Autodesk Fusion 360 part; units mm, degrees
(part 2 of 14)
  line L872 (-87.0011, -128.5875) -> (-81.5018, -138.1125)
  line L873 (-81.5018, -119.0625) -> (-87.0011, -128.5875)
  line L874 (-100.7493, -149.225) -> (-89.7507, -149.225)
  line L875 (-89.7507, -149.225) -> (-84.2515, -139.7)
  line L876 (-84.2515, -139.7) -> (-89.7507, -130.175)
  line L877 (-89.7507, -130.175) -> (-100.7493, -130.175)
  line L878 (-106.2485, -139.7) -> (-100.7493, -149.225)
  line L879 (-100.7493, -130.175) -> (-106.2485, -139.7)
  line L880 (-119.9967, -160.3375) -> (-108.9982, -160.3375)
  line L881 (-108.9982, -160.3375) -> (-103.4989, -150.8125)
  line L882 (-103.4989, -150.8125) -> (-108.9982, -141.2875)
  line L883 (-108.9982, -141.2875) -> (-119.9967, -141.2875)
  line L884 (-125.4959, -150.8125) -> (-119.9967, -160.3375)
  line L885 (-119.9967, -141.2875) -> (-125.4959, -150.8125)
  line L886 (-139.2441, -171.45) -> (-128.2456, -171.45)
  line L887 (-128.2456, -171.45) -> (-122.7463, -161.925)
  line L888 (-122.7463, -161.925) -> (-128.2456, -152.4)
  line L889 (-128.2456, -152.4) -> (-139.2441, -152.4)
  line L890 (-144.7434, -161.925) -> (-139.2441, -171.45)
  line L891 (-139.2441, -152.4) -> (-144.7434, -161.925)
  line L892 (-158.4915, -182.5625) -> (-147.493, -182.5625)
  line L893 (-147.493, -182.5625) -> (-141.9937, -173.0375)
  line L894 (-141.9937, -173.0375) -> (-147.493, -163.5125)
  line L895 (-147.493, -163.5125) -> (-158.4915, -163.5125)
  line L896 (-163.9908, -173.0375) -> (-158.4915, -182.5625)
  line L897 (-158.4915, -163.5125) -> (-163.9908, -173.0375)
  line L898 (-177.7389, -193.675) -> (-166.7404, -193.675)
  line L899 (-166.7404, -193.675) -> (-161.2411, -184.15)
  line L900 (-161.2411, -184.15) -> (-166.7404, -174.625)
  line L901 (-166.7404, -174.625) -> (-177.7389, -174.625)
  line L902 (-183.2382, -184.15) -> (-177.7389, -193.675)
  line L903 (-177.7389, -174.625) -> (-183.2382, -184.15)
  line L904 (-196.9863, -204.7875) -> (-185.9878, -204.7875)
  line L905 (-185.9878, -204.7875) -> (-180.4886, -195.2625)
  line L906 (-180.4886, -195.2625) -> (-185.9878, -185.7375)
  line L907 (-185.9878, -185.7375) -> (-196.9863, -185.7375)
  line L908 (-202.4856, -195.2625) -> (-196.9863, -204.7875)
  line L909 (-196.9863, -185.7375) -> (-202.4856, -195.2625)
  line L910 (91.7249, -60.325) -> (102.7234, -60.325)
  line L911 (102.7234, -60.325) -> (108.2227, -50.8)
  line L912 (108.2227, -50.8) -> (102.7234, -41.275)
  line L913 (102.7234, -41.275) -> (91.7249, -41.275)
  line L914 (86.2256, -50.8) -> (91.7249, -60.325)
  line L915 (91.7249, -41.275) -> (86.2256, -50.8)
  line L916 (72.4775, -71.4375) -> (83.476, -71.4375)
  line L917 (83.476, -71.4375) -> (88.9753, -61.9125)
  line L918 (88.9753, -61.9125) -> (83.476, -52.3875)
  line L919 (83.476, -52.3875) -> (72.4775, -52.3875)
  line L920 (66.9782, -61.9125) -> (72.4775, -71.4375)
  line L921 (72.4775, -52.3875) -> (66.9782, -61.9125)
  line L922 (53.2301, -82.55) -> (64.2286, -82.55)
  line L923 (64.2286, -82.55) -> (69.7278, -73.025)
  line L924 (69.7278, -73.025) -> (64.2286, -63.5)
  line L925 (64.2286, -63.5) -> (53.2301, -63.5)
  line L926 (47.7308, -73.025) -> (53.2301, -82.55)
  line L927 (53.2301, -63.5) -> (47.7308, -73.025)
  line L928 (33.9826, -93.6625) -> (44.9812, -93.6625)
  line L929 (44.9812, -93.6625) -> (50.4804, -84.1375)
  line L930 (50.4804, -84.1375) -> (44.9812, -74.6125)
  line L931 (44.9812, -74.6125) -> (33.9826, -74.6125)
  line L932 (28.4834, -84.1375) -> (33.9826, -93.6625)
  line L933 (33.9826, -74.6125) -> (28.4834, -84.1375)
  line L934 (14.7352, -104.775) -> (25.7337, -104.775)
  line L935 (25.7337, -104.775) -> (31.233, -95.25)
  line L936 (31.233, -95.25) -> (25.7337, -85.725)
  line L937 (25.7337, -85.725) -> (14.7352, -85.725)
  line L938 (9.236, -95.25) -> (14.7352, -104.775)
  line L939 (14.7352, -85.725) -> (9.236, -95.25)
  line L940 (-4.5122, -115.8875) -> (6.4863, -115.8875)
  line L941 (6.4863, -115.8875) -> (11.9856, -106.3625)
  line L942 (11.9856, -106.3625) -> (6.4863, -96.8375)
  line L943 (6.4863, -96.8375) -> (-4.5122, -96.8375)
  line L944 (-10.0114, -106.3625) -> (-4.5122, -115.8875)
  line L945 (-4.5122, -96.8375) -> (-10.0114, -106.3625)
  line L946 (-23.7596, -127) -> (-12.7611, -127)
  line L947 (-12.7611, -127) -> (-7.2618, -117.475)
  line L948 (-7.2618, -117.475) -> (-12.7611, -107.95)
  line L949 (-12.7611, -107.95) -> (-23.7596, -107.95)
  line L950 (-29.2589, -117.475) -> (-23.7596, -127)
  line L951 (-23.7596, -107.95) -> (-29.2589, -117.475)
  line L952 (-43.007, -138.1125) -> (-32.0085, -138.1125)
  line L953 (-32.0085, -138.1125) -> (-26.5092, -128.5875)
  line L954 (-26.5092, -128.5875) -> (-32.0085, -119.0625)
  line L955 (-32.0085, -119.0625) -> (-43.007, -119.0625)
  line L956 (-48.5063, -128.5875) -> (-43.007, -138.1125)
  line L957 (-43.007, -119.0625) -> (-48.5063, -128.5875)
  line L958 (-62.2544, -149.225) -> (-51.2559, -149.225)
  line L959 (-51.2559, -149.225) -> (-45.7566, -139.7)
  line L960 (-45.7566, -139.7) -> (-51.2559, -130.175)
  line L961 (-51.2559, -130.175) -> (-62.2544, -130.175)
  line L962 (-67.7537, -139.7) -> (-62.2544, -149.225)
  line L963 (-62.2544, -130.175) -> (-67.7537, -139.7)
  line L964 (-81.5018, -160.3375) -> (-70.5033, -160.3375)
  line L965 (-70.5033, -160.3375) -> (-65.0041, -150.8125)
  line L966 (-65.0041, -150.8125) -> (-70.5033, -141.2875)
  line L967 (-70.5033, -141.2875) -> (-81.5018, -141.2875)
  line L968 (-87.0011, -150.8125) -> (-81.5018, -160.3375)
  line L969 (-81.5018, -141.2875) -> (-87.0011, -150.8125)
  line L970 (-100.7493, -171.45) -> (-89.7507, -171.45)
  line L971 (-89.7507, -171.45) -> (-84.2515, -161.925)
  line L972 (-84.2515, -161.925) -> (-89.7507, -152.4)
  line L973 (-89.7507, -152.4) -> (-100.7493, -152.4)
  line L974 (-106.2485, -161.925) -> (-100.7493, -171.45)
  line L975 (-100.7493, -152.4) -> (-106.2485, -161.925)
  line L976 (-119.9967, -182.5625) -> (-108.9982, -182.5625)
  line L977 (-108.9982, -182.5625) -> (-103.4989, -173.0375)
  line L978 (-103.4989, -173.0375) -> (-108.9982, -163.5125)
  line L979 (-108.9982, -163.5125) -> (-119.9967, -163.5125)
  line L980 (-125.4959, -173.0375) -> (-119.9967, -182.5625)
  line L981 (-119.9967, -163.5125) -> (-125.4959, -173.0375)
  line L982 (-139.2441, -193.675) -> (-128.2456, -193.675)
  line L983 (-128.2456, -193.675) -> (-122.7463, -184.15)
  line L984 (-122.7463, -184.15) -> (-128.2456, -174.625)
  line L985 (-128.2456, -174.625) -> (-139.2441, -174.625)
  line L986 (-144.7434, -184.15) -> (-139.2441, -193.675)
  line L987 (-139.2441, -174.625) -> (-144.7434, -184.15)
  line L988 (-158.4915, -204.7875) -> (-147.493, -204.7875)
  line L989 (-147.493, -204.7875) -> (-141.9937, -195.2625)
  line L990 (-141.9937, -195.2625) -> (-147.493, -185.7375)
  line L991 (-147.493, -185.7375) -> (-158.4915, -185.7375)
  line L992 (-163.9908, -195.2625) -> (-158.4915, -204.7875)
  line L993 (-158.4915, -185.7375) -> (-163.9908, -195.2625)
  line L994 (-177.7389, -215.9) -> (-166.7404, -215.9)
  line L995 (-166.7404, -215.9) -> (-161.2411, -206.375)
  line L996 (-161.2411, -206.375) -> (-166.7404, -196.85)
  line L997 (-166.7404, -196.85) -> (-177.7389, -196.85)
  line L998 (-183.2382, -206.375) -> (-177.7389, -215.9)
  line L999 (-177.7389, -196.85) -> (-183.2382, -206.375)
  line L1000 (110.9723, -71.4375) -> (121.9708, -71.4375)
  line L1001 (121.9708, -71.4375) -> (127.4701, -61.9125)
  line L1002 (127.4701, -61.9125) -> (121.9708, -52.3875)
  line L1003 (121.9708, -52.3875) -> (110.9723, -52.3875)
  line L1004 (105.473, -61.9125) -> (110.9723, -71.4375)
  line L1005 (110.9723, -52.3875) -> (105.473, -61.9125)
  line L1006 (91.7249, -82.55) -> (102.7234, -82.55)
  line L1007 (102.7234, -82.55) -> (108.2227, -73.025)
  line L1008 (108.2227, -73.025) -> (102.7234, -63.5)
  line L1009 (102.7234, -63.5) -> (91.7249, -63.5)
  line L1010 (86.2256, -73.025) -> (91.7249, -82.55)
  line L1011 (91.7249, -63.5) -> (86.2256, -73.025)
  line L1012 (72.4775, -93.6625) -> (83.476, -93.6625)
  line L1013 (83.476, -93.6625) -> (88.9753, -84.1375)
  line L1014 (88.9753, -84.1375) -> (83.476, -74.6125)
  line L1015 (83.476, -74.6125) -> (72.4775, -74.6125)
  line L1016 (66.9782, -84.1375) -> (72.4775, -93.6625)
  line L1017 (72.4775, -74.6125) -> (66.9782, -84.1375)
  line L1018 (53.2301, -104.775) -> (64.2286, -104.775)
  line L1019 (64.2286, -104.775) -> (69.7278, -95.25)
  line L1020 (69.7278, -95.25) -> (64.2286, -85.725)
  line L1021 (64.2286, -85.725) -> (53.2301, -85.725)
  line L1022 (47.7308, -95.25) -> (53.2301, -104.775)
  line L1023 (53.2301, -85.725) -> (47.7308, -95.25)
  line L1024 (33.9826, -115.8875) -> (44.9812, -115.8875)
  line L1025 (44.9812, -115.8875) -> (50.4804, -106.3625)
  line L1026 (50.4804, -106.3625) -> (44.9812, -96.8375)
  line L1027 (44.9812, -96.8375) -> (33.9826, -96.8375)
  line L1028 (28.4834, -106.3625) -> (33.9826, -115.8875)
  line L1029 (33.9826, -96.8375) -> (28.4834, -106.3625)
  line L1030 (14.7352, -127) -> (25.7337, -127)
  line L1031 (25.7337, -127) -> (31.233, -117.475)
  line L1032 (31.233, -117.475) -> (25.7337, -107.95)
  line L1033 (25.7337, -107.95) -> (14.7352, -107.95)
  line L1034 (9.236, -117.475) -> (14.7352, -127)
  line L1035 (14.7352, -107.95) -> (9.236, -117.475)
  line L1036 (-4.5122, -138.1125) -> (6.4863, -138.1125)
  line L1037 (6.4863, -138.1125) -> (11.9856, -128.5875)
  line L1038 (11.9856, -128.5875) -> (6.4863, -119.0625)
  line L1039 (6.4863, -119.0625) -> (-4.5122, -119.0625)
  line L1040 (-10.0114, -128.5875) -> (-4.5122, -138.1125)
  line L1041 (-4.5122, -119.0625) -> (-10.0114, -128.5875)
  line L1042 (-23.7596, -149.225) -> (-12.7611, -149.225)
  line L1043 (-12.7611, -149.225) -> (-7.2618, -139.7)
  line L1044 (-7.2618, -139.7) -> (-12.7611, -130.175)
  line L1045 (-12.7611, -130.175) -> (-23.7596, -130.175)
  line L1046 (-29.2589, -139.7) -> (-23.7596, -149.225)
  line L1047 (-23.7596, -130.175) -> (-29.2589, -139.7)
  line L1048 (-43.007, -160.3375) -> (-32.0085, -160.3375)
  line L1049 (-32.0085, -160.3375) -> (-26.5092, -150.8125)
  line L1050 (-26.5092, -150.8125) -> (-32.0085, -141.2875)
  line L1051 (-32.0085, -141.2875) -> (-43.007, -141.2875)
  line L1052 (-48.5063, -150.8125) -> (-43.007, -160.3375)
  line L1053 (-43.007, -141.2875) -> (-48.5063, -150.8125)
  line L1054 (-62.2544, -171.45) -> (-51.2559, -171.45)
  line L1055 (-51.2559, -171.45) -> (-45.7566, -161.925)
  line L1056 (-45.7566, -161.925) -> (-51.2559, -152.4)
  line L1057 (-51.2559, -152.4) -> (-62.2544, -152.4)
  line L1058 (-67.7537, -161.925) -> (-62.2544, -171.45)
  line L1059 (-62.2544, -152.4) -> (-67.7537, -161.925)
  line L1060 (-81.5018, -182.5625) -> (-70.5033, -182.5625)
  line L1061 (-70.5033, -182.5625) -> (-65.0041, -173.0375)
  line L1062 (-65.0041, -173.0375) -> (-70.5033, -163.5125)
  line L1063 (-70.5033, -163.5125) -> (-81.5018, -163.5125)
  line L1064 (-87.0011, -173.0375) -> (-81.5018, -182.5625)
  line L1065 (-81.5018, -163.5125) -> (-87.0011, -173.0375)
  line L1066 (-100.7493, -193.675) -> (-89.7507, -193.675)
  line L1067 (-89.7507, -193.675) -> (-84.2515, -184.15)
  line L1068 (-84.2515, -184.15) -> (-89.7507, -174.625)
  line L1069 (-89.7507, -174.625) -> (-100.7493, -174.625)
  line L1070 (-106.2485, -184.15) -> (-100.7493, -193.675)
  line L1071 (-100.7493, -174.625) -> (-106.2485, -184.15)
  line L1072 (-119.9967, -204.7875) -> (-108.9982, -204.7875)
  line L1073 (-108.9982, -204.7875) -> (-103.4989, -195.2625)
  line L1074 (-103.4989, -195.2625) -> (-108.9982, -185.7375)
  line L1075 (-108.9982, -185.7375) -> (-119.9967, -185.7375)
  line L1076 (-125.4959, -195.2625) -> (-119.9967, -204.7875)
  line L1077 (-119.9967, -185.7375) -> (-125.4959, -195.2625)
  line L1078 (-139.2441, -215.9) -> (-128.2456, -215.9)
  line L1079 (-128.2456, -215.9) -> (-122.7463, -206.375)
  line L1080 (-122.7463, -206.375) -> (-128.2456, -196.85)
  line L1081 (-128.2456, -196.85) -> (-139.2441, -196.85)
  line L1082 (-144.7434, -206.375) -> (-139.2441, -215.9)
  line L1083 (-139.2441, -196.85) -> (-144.7434, -206.375)
  line L1084 (-158.4915, -227.0125) -> (-147.493, -227.0125)
  line L1085 (-147.493, -227.0125) -> (-141.9937, -217.4875)
  line L1086 (-141.9937, -217.4875) -> (-147.493, -207.9625)
  line L1087 (-147.493, -207.9625) -> (-158.4915, -207.9625)
  line L1088 (-163.9908, -217.4875) -> (-158.4915, -227.0125)
  line L1089 (-158.4915, -207.9625) -> (-163.9908, -217.4875)
  line L1090 (130.2197, -82.55) -> (141.2182, -82.55)
  line L1091 (141.2182, -82.55) -> (146.7175, -73.025)
  line L1092 (146.7175, -73.025) -> (141.2182, -63.5)
  line L1093 (141.2182, -63.5) -> (130.2197, -63.5)
  line L1094 (124.7205, -73.025) -> (130.2197, -82.55)
  line L1095 (130.2197, -63.5) -> (124.7205, -73.025)
  line L1096 (110.9723, -93.6625) -> (121.9708, -93.6625)
  line L1097 (121.9708, -93.6625) -> (127.4701, -84.1375)
  line L1098 (127.4701, -84.1375) -> (121.9708, -74.6125)
  line L1099 (121.9708, -74.6125) -> (110.9723, -74.6125)
  line L1100 (105.473, -84.1375) -> (110.9723, -93.6625)
  line L1101 (110.9723, -74.6125) -> (105.473, -84.1375)
  line L1102 (91.7249, -104.775) -> (102.7234, -104.775)
  line L1103 (102.7234, -104.775) -> (108.2227, -95.25)
  line L1104 (108.2227, -95.25) -> (102.7234, -85.725)
  line L1105 (102.7234, -85.725) -> (91.7249, -85.725)
  line L1106 (86.2256, -95.25) -> (91.7249, -104.775)
  line L1107 (91.7249, -85.725) -> (86.2256, -95.25)
  line L1108 (72.4775, -115.8875) -> (83.476, -115.8875)
  line L1109 (83.476, -115.8875) -> (88.9753, -106.3625)
  line L1110 (88.9753, -106.3625) -> (83.476, -96.8375)
  line L1111 (83.476, -96.8375) -> (72.4775, -96.8375)
  line L1112 (66.9782, -106.3625) -> (72.4775, -115.8875)
  line L1113 (72.4775, -96.8375) -> (66.9782, -106.3625)
  line L1114 (53.2301, -127) -> (64.2286, -127)
  line L1115 (64.2286, -127) -> (69.7278, -117.475)
  line L1116 (69.7278, -117.475) -> (64.2286, -107.95)
  line L1117 (64.2286, -107.95) -> (53.2301, -107.95)
  line L1118 (47.7308, -117.475) -> (53.2301, -127)
  line L1119 (53.2301, -107.95) -> (47.7308, -117.475)
  line L1120 (33.9826, -138.1125) -> (44.9812, -138.1125)
  line L1121 (44.9812, -138.1125) -> (50.4804, -128.5875)
  line L1122 (50.4804, -128.5875) -> (44.9812, -119.0625)
  line L1123 (44.9812, -119.0625) -> (33.9826, -119.0625)
  line L1124 (28.4834, -128.5875) -> (33.9826, -138.1125)
  line L1125 (33.9826, -119.0625) -> (28.4834, -128.5875)
  line L1126 (14.7352, -149.225) -> (25.7337, -149.225)
  line L1127 (25.7337, -149.225) -> (31.233, -139.7)
  line L1128 (31.233, -139.7) -> (25.7337, -130.175)
  line L1129 (25.7337, -130.175) -> (14.7352, -130.175)
  line L1130 (9.236, -139.7) -> (14.7352, -149.225)
  line L1131 (14.7352, -130.175) -> (9.236, -139.7)
  line L1132 (-4.5122, -160.3375) -> (6.4863, -160.3375)
  line L1133 (6.4863, -160.3375) -> (11.9856, -150.8125)
  line L1134 (11.9856, -150.8125) -> (6.4863, -141.2875)
  line L1135 (6.4863, -141.2875) -> (-4.5122, -141.2875)
  line L1136 (-10.0114, -150.8125) -> (-4.5122, -160.3375)
  line L1137 (-4.5122, -141.2875) -> (-10.0114, -150.8125)
  line L1138 (-23.7596, -171.45) -> (-12.7611, -171.45)
  line L1139 (-12.7611, -171.45) -> (-7.2618, -161.925)
  line L1140 (-7.2618, -161.925) -> (-12.7611, -152.4)
  line L1141 (-12.7611, -152.4) -> (-23.7596, -152.4)
  line L1142 (-29.2589, -161.925) -> (-23.7596, -171.45)
  line L1143 (-23.7596, -152.4) -> (-29.2589, -161.925)
  line L1144 (-43.007, -182.5625) -> (-32.0085, -182.5625)
  line L1145 (-32.0085, -182.5625) -> (-26.5092, -173.0375)
  line L1146 (-26.5092, -173.0375) -> (-32.0085, -163.5125)
  line L1147 (-32.0085, -163.5125) -> (-43.007, -163.5125)
  line L1148 (-48.5063, -173.0375) -> (-43.007, -182.5625)
  line L1149 (-43.007, -163.5125) -> (-48.5063, -173.0375)
  line L1150 (-62.2544, -193.675) -> (-51.2559, -193.675)
  line L1151 (-51.2559, -193.675) -> (-45.7566, -184.15)
  line L1152 (-45.7566, -184.15) -> (-51.2559, -174.625)
  line L1153 (-51.2559, -174.625) -> (-62.2544, -174.625)
  line L1154 (-67.7537, -184.15) -> (-62.2544, -193.675)
  line L1155 (-62.2544, -174.625) -> (-67.7537, -184.15)
  line L1156 (-81.5018, -204.7875) -> (-70.5033, -204.7875)
  line L1157 (-70.5033, -204.7875) -> (-65.0041, -195.2625)
  line L1158 (-65.0041, -195.2625) -> (-70.5033, -185.7375)
  line L1159 (-70.5033, -185.7375) -> (-81.5018, -185.7375)
  line L1160 (-87.0011, -195.2625) -> (-81.5018, -204.7875)
  line L1161 (-81.5018, -185.7375) -> (-87.0011, -195.2625)
  line L1162 (-100.7493, -215.9) -> (-89.7507, -215.9)
  line L1163 (-89.7507, -215.9) -> (-84.2515, -206.375)
  line L1164 (-84.2515, -206.375) -> (-89.7507, -196.85)
  line L1165 (-89.7507, -196.85) -> (-100.7493, -196.85)
  line L1166 (-106.2485, -206.375) -> (-100.7493, -215.9)
  line L1167 (-100.7493, -196.85) -> (-106.2485, -206.375)
  line L1168 (-119.9967, -227.0125) -> (-108.9982, -227.0125)
  line L1169 (-108.9982, -227.0125) -> (-103.4989, -217.4875)
  line L1170 (-103.4989, -217.4875) -> (-108.9982, -207.9625)
  line L1171 (-108.9982, -207.9625) -> (-119.9967, -207.9625)
  line L1172 (-125.4959, -217.4875) -> (-119.9967, -227.0125)
  line L1173 (-119.9967, -207.9625) -> (-125.4959, -217.4875)
  line L1174 (-139.2441, -238.125) -> (-128.2456, -238.125)
  line L1175 (-128.2456, -238.125) -> (-122.7463, -228.6)
  line L1176 (-122.7463, -228.6) -> (-128.2456, -219.075)
  line L1177 (-128.2456, -219.075) -> (-139.2441, -219.075)
  line L1178 (-144.7434, -228.6) -> (-139.2441, -238.125)
  line L1179 (-139.2441, -219.075) -> (-144.7434, -228.6)
  line L1180 (149.4671, -93.6625) -> (160.4657, -93.6625)
  line L1181 (160.4657, -93.6625) -> (165.9649, -84.1375)
  line L1182 (165.9649, -84.1375) -> (160.4657, -74.6125)
  line L1183 (160.4657, -74.6125) -> (149.4671, -74.6125)
  line L1184 (143.9679, -84.1375) -> (149.4671, -93.6625)
  line L1185 (149.4671, -74.6125) -> (143.9679, -84.1375)
  line L1186 (130.2197, -104.775) -> (141.2182, -104.775)
  line L1187 (141.2182, -104.775) -> (146.7175, -95.25)
  line L1188 (146.7175, -95.25) -> (141.2182, -85.725)
  line L1189 (141.2182, -85.725) -> (130.2197, -85.725)
  line L1190 (124.7205, -95.25) -> (130.2197, -104.775)
  line L1191 (130.2197, -85.725) -> (124.7205, -95.25)
  line L1192 (110.9723, -115.8875) -> (121.9708, -115.8875)
  line L1193 (121.9708, -115.8875) -> (127.4701, -106.3625)
  line L1194 (127.4701, -106.3625) -> (121.9708, -96.8375)
  line L1195 (121.9708, -96.8375) -> (110.9723, -96.8375)
  line L1196 (105.473, -106.3625) -> (110.9723, -115.8875)
  line L1197 (110.9723, -96.8375) -> (105.473, -106.3625)
  line L1198 (91.7249, -127) -> (102.7234, -127)
  line L1199 (102.7234, -127) -> (108.2227, -117.475)
  line L1200 (108.2227, -117.475) -> (102.7234, -107.95)
  line L1201 (102.7234, -107.95) -> (91.7249, -107.95)
  line L1202 (86.2256, -117.475) -> (91.7249, -127)
  line L1203 (91.7249, -107.95) -> (86.2256, -117.475)
  line L1204 (72.4775, -138.1125) -> (83.476, -138.1125)
  line L1205 (83.476, -138.1125) -> (88.9753, -128.5875)
  line L1206 (88.9753, -128.5875) -> (83.476, -119.0625)
  line L1207 (83.476, -119.0625) -> (72.4775, -119.0625)
  line L1208 (66.9782, -128.5875) -> (72.4775, -138.1125)
  line L1209 (72.4775, -119.0625) -> (66.9782, -128.5875)
  line L1210 (53.2301, -149.225) -> (64.2286, -149.225)
  line L1211 (64.2286, -149.225) -> (69.7278, -139.7)
  line L1212 (69.7278, -139.7) -> (64.2286, -130.175)
  line L1213 (64.2286, -130.175) -> (53.2301, -130.175)
  line L1214 (47.7308, -139.7) -> (53.2301, -149.225)
  line L1215 (53.2301, -130.175) -> (47.7308, -139.7)
  line L1216 (33.9826, -160.3375) -> (44.9812, -160.3375)
  line L1217 (44.9812, -160.3375) -> (50.4804, -150.8125)
  line L1218 (50.4804, -150.8125) -> (44.9812, -141.2875)
  line L1219 (44.9812, -141.2875) -> (33.9826, -141.2875)
  line L1220 (28.4834, -150.8125) -> (33.9826, -160.3375)
  line L1221 (33.9826, -141.2875) -> (28.4834, -150.8125)
  line L1222 (14.7352, -171.45) -> (25.7337, -171.45)
  line L1223 (25.7337, -171.45) -> (31.233, -161.925)
  line L1224 (31.233, -161.925) -> (25.7337, -152.4)
  line L1225 (25.7337, -152.4) -> (14.7352, -152.4)
  line L1226 (9.236, -161.925) -> (14.7352, -171.45)
  line L1227 (14.7352, -152.4) -> (9.236, -161.925)
  line L1228 (-4.5122, -182.5625) -> (6.4863, -182.5625)
  line L1229 (6.4863, -182.5625) -> (11.9856, -173.0375)
  line L1230 (11.9856, -173.0375) -> (6.4863, -163.5125)
  line L1231 (6.4863, -163.5125) -> (-4.5122, -163.5125)
  line L1232 (-10.0114, -173.0375) -> (-4.5122, -182.5625)
  line L1233 (-4.5122, -163.5125) -> (-10.0114, -173.0375)
  line L1234 (-23.7596, -193.675) -> (-12.7611, -193.675)
  line L1235 (-12.7611, -193.675) -> (-7.2618, -184.15)
  line L1236 (-7.2618, -184.15) -> (-12.7611, -174.625)
  line L1237 (-12.7611, -174.625) -> (-23.7596, -174.625)
  line L1238 (-29.2589, -184.15) -> (-23.7596, -193.675)
  line L1239 (-23.7596, -174.625) -> (-29.2589, -184.15)
  line L1240 (-43.007, -204.7875) -> (-32.0085, -204.7875)
  line L1241 (-32.0085, -204.7875) -> (-26.5092, -195.2625)
  line L1242 (-26.5092, -195.2625) -> (-32.0085, -185.7375)
  line L1243 (-32.0085, -185.7375) -> (-43.007, -185.7375)
  line L1244 (-48.5063, -195.2625) -> (-43.007, -204.7875)
  line L1245 (-43.007, -185.7375) -> (-48.5063, -195.2625)
  line L1246 (-62.2544, -215.9) -> (-51.2559, -215.9)
  line L1247 (-51.2559, -215.9) -> (-45.7566, -206.375)
  line L1248 (-45.7566, -206.375) -> (-51.2559, -196.85)
  line L1249 (-51.2559, -196.85) -> (-62.2544, -196.85)
  line L1250 (-67.7537, -206.375) -> (-62.2544, -215.9)
  line L1251 (-62.2544, -196.85) -> (-67.7537, -206.375)
  line L1252 (-81.5018, -227.0125) -> (-70.5033, -227.0125)
  line L1253 (-70.5033, -227.0125) -> (-65.0041, -217.4875)
  line L1254 (-65.0041, -217.4875) -> (-70.5033, -207.9625)
  line L1255 (-70.5033, -207.9625) -> (-81.5018, -207.9625)
  line L1256 (-87.0011, -217.4875) -> (-81.5018, -227.0125)
  line L1257 (-81.5018, -207.9625) -> (-87.0011, -217.4875)
  line L1258 (-100.7493, -238.125) -> (-89.7507, -238.125)
  line L1259 (-89.7507, -238.125) -> (-84.2515, -228.6)
  line L1260 (-84.2515, -228.6) -> (-89.7507, -219.075)
  line L1261 (-89.7507, -219.075) -> (-100.7493, -219.075)
  line L1262 (-106.2485, -228.6) -> (-100.7493, -238.125)
  line L1263 (-100.7493, -219.075) -> (-106.2485, -228.6)
  line L1264 (-119.9967, -249.2375) -> (-108.9982, -249.2375)
  line L1265 (-108.9982, -249.2375) -> (-103.4989, -239.7125)
  line L1266 (-103.4989, -239.7125) -> (-108.9982, -230.1875)
  line L1267 (-108.9982, -230.1875) -> (-119.9967, -230.1875)
  line L1268 (-125.4959, -239.7125) -> (-119.9967, -249.2375)
  line L1269 (-119.9967, -230.1875) -> (-125.4959, -239.7125)
  line L1270 (168.7145, -104.775) -> (179.7131, -104.775)
  line L1271 (179.7131, -104.775) -> (185.2123, -95.25)
  line L1272 (185.2123, -95.25) -> (179.7131, -85.725)
  line L1273 (179.7131, -85.725) -> (168.7145, -85.725)
  line L1274 (163.2153, -95.25) -> (168.7145, -104.775)
  line L1275 (168.7145, -85.725) -> (163.2153, -95.25)
  line L1276 (149.4671, -115.8875) -> (160.4657, -115.8875)
  line L1277 (160.4657, -115.8875) -> (165.9649, -106.3625)
  line L1278 (165.9649, -106.3625) -> (160.4657, -96.8375)
  line L1279 (160.4657, -96.8375) -> (149.4671, -96.8375)
  line L1280 (143.9679, -106.3625) -> (149.4671, -115.8875)
  line L1281 (149.4671, -96.8375) -> (143.9679, -106.3625)
  line L1282 (130.2197, -127) -> (141.2182, -127)
  line L1283 (141.2182, -127) -> (146.7175, -117.475)
  line L1284 (146.7175, -117.475) -> (141.2182, -107.95)
  line L1285 (141.2182, -107.95) -> (130.2197, -107.95)
  line L1286 (124.7205, -117.475) -> (130.2197, -127)
  line L1287 (130.2197, -107.95) -> (124.7205, -117.475)
  line L1288 (110.9723, -138.1125) -> (121.9708, -138.1125)
  line L1289 (121.9708, -138.1125) -> (127.4701, -128.5875)
  line L1290 (127.4701, -128.5875) -> (121.9708, -119.0625)
  line L1291 (121.9708, -119.0625) -> (110.9723, -119.0625)
  line L1292 (105.473, -128.5875) -> (110.9723, -138.1125)
  line L1293 (110.9723, -119.0625) -> (105.473, -128.5875)
  line L1294 (91.7249, -149.225) -> (102.7234, -149.225)
  line L1295 (102.7234, -149.225) -> (108.2227, -139.7)
  line L1296 (108.2227, -139.7) -> (102.7234, -130.175)
  line L1297 (102.7234, -130.175) -> (91.7249, -130.175)
  line L1298 (86.2256, -139.7) -> (91.7249, -149.225)
  line L1299 (91.7249, -130.175) -> (86.2256, -139.7)
  line L1300 (72.4775, -160.3375) -> (83.476, -160.3375)
  line L1301 (83.476, -160.3375) -> (88.9753, -150.8125)
  line L1302 (88.9753, -150.8125) -> (83.476, -141.2875)
  line L1303 (83.476, -141.2875) -> (72.4775, -141.2875)
  line L1304 (66.9782, -150.8125) -> (72.4775, -160.3375)
  line L1305 (72.4775, -141.2875) -> (66.9782, -150.8125)
  line L1306 (53.2301, -171.45) -> (64.2286, -171.45)
  line L1307 (64.2286, -171.45) -> (69.7278, -161.925)
  line L1308 (69.7278, -161.925) -> (64.2286, -152.4)
  line L1309 (64.2286, -152.4) -> (53.2301, -152.4)
  line L1310 (47.7308, -161.925) -> (53.2301, -171.45)
  line L1311 (53.2301, -152.4) -> (47.7308, -161.925)
  line L1312 (33.9826, -182.5625) -> (44.9812, -182.5625)
  line L1313 (44.9812, -182.5625) -> (50.4804, -173.0375)
  line L1314 (50.4804, -173.0375) -> (44.9812, -163.5125)
  line L1315 (44.9812, -163.5125) -> (33.9826, -163.5125)
  line L1316 (28.4834, -173.0375) -> (33.9826, -182.5625)
  line L1317 (33.9826, -163.5125) -> (28.4834, -173.0375)
  line L1318 (14.7352, -193.675) -> (25.7337, -193.675)
  line L1319 (25.7337, -193.675) -> (31.233, -184.15)
  line L1320 (31.233, -184.15) -> (25.7337, -174.625)
  line L1321 (25.7337, -174.625) -> (14.7352, -174.625)
  line L1322 (9.236, -184.15) -> (14.7352, -193.675)
  line L1323 (14.7352, -174.625) -> (9.236, -184.15)
  line L1324 (-4.5122, -204.7875) -> (6.4863, -204.7875)
  line L1325 (6.4863, -204.7875) -> (11.9856, -195.2625)
  line L1326 (11.9856, -195.2625) -> (6.4863, -185.7375)
  line L1327 (6.4863, -185.7375) -> (-4.5122, -185.7375)
  line L1328 (-10.0114, -195.2625) -> (-4.5122, -204.7875)
  line L1329 (-4.5122, -185.7375) -> (-10.0114, -195.2625)
  line L1330 (-23.7596, -215.9) -> (-12.7611, -215.9)
  line L1331 (-12.7611, -215.9) -> (-7.2618, -206.375)
  line L1332 (-7.2618, -206.375) -> (-12.7611, -196.85)
  line L1333 (-12.7611, -196.85) -> (-23.7596, -196.85)
  line L1334 (-29.2589, -206.375) -> (-23.7596, -215.9)
  line L1335 (-23.7596, -196.85) -> (-29.2589, -206.375)
  line L1336 (-43.007, -227.0125) -> (-32.0085, -227.0125)
  line L1337 (-32.0085, -227.0125) -> (-26.5092, -217.4875)
  line L1338 (-26.5092, -217.4875) -> (-32.0085, -207.9625)
  line L1339 (-32.0085, -207.9625) -> (-43.007, -207.9625)
  line L1340 (-48.5063, -217.4875) -> (-43.007, -227.0125)
  line L1341 (-43.007, -207.9625) -> (-48.5063, -217.4875)
  line L1342 (-62.2544, -238.125) -> (-51.2559, -238.125)
  line L1343 (-51.2559, -238.125) -> (-45.7566, -228.6)
  line L1344 (-45.7566, -228.6) -> (-51.2559, -219.075)
  line L1345 (-51.2559, -219.075) -> (-62.2544, -219.075)
  line L1346 (-67.7537, -228.6) -> (-62.2544, -238.125)
  line L1347 (-62.2544, -219.075) -> (-67.7537, -228.6)
  line L1348 (-81.5018, -249.2375) -> (-70.5033, -249.2375)
  line L1349 (-70.5033, -249.2375) -> (-65.0041, -239.7125)
  line L1350 (-65.0041, -239.7125) -> (-70.5033, -230.1875)
  line L1351 (-70.5033, -230.1875) -> (-81.5018, -230.1875)
  line L1352 (-87.0011, -239.7125) -> (-81.5018, -249.2375)
  line L1353 (-81.5018, -230.1875) -> (-87.0011, -239.7125)
  line L1354 (-100.7493, -260.35) -> (-89.7507, -260.35)
  line L1355 (-89.7507, -260.35) -> (-84.2515, -250.825)
  line L1356 (-84.2515, -250.825) -> (-89.7507, -241.3)
  line L1357 (-89.7507, -241.3) -> (-100.7493, -241.3)
  line L1358 (-106.2485, -250.825) -> (-100.7493, -260.35)
  line L1359 (-100.7493, -241.3) -> (-106.2485, -250.825)
  point P0 (-95.25, -95.25)
  dimension "d8" = 9.525
  dimension "d9" = 120
  dimension "d13" = 22.225
  dimension "d14" = 22.225
  constraint coincident L1.end L2.start
  constraint coincident L0.start L3.end
  constraint coincident L2.end L3.start
  constraint coincident L0.end L1.start
  constraint midpoint L4 P0
  constraint horizontal L13
  constraint coincident P0 L12.start
  constraint coincident L6.start L12
  constraint midpoint L11 L14.end
  constraint midpoint L7 L15.end
  measures "d8" distance of P0 L11
  measures "d9" angle of L12 L13
extrude "Extrude3" cut sketch "Sketch2" against normal blind 6.35 contours L0 L1 L2 L3 L46 L47 L130 L131 L134 L136 L137 L138 L140 L141 L142 L143 L144 L145 L214 L215 L218 L220 L221 L222 L224 L225 L238 L239 L240 L241 L298 L299 L302 L304 L305 L306 L308 L309 L334 L335 L336 L337 L382 L383 L386 L388 L389 L390 L392 L393 L430 L431 L432 L433 L466 L470 L472 L473 L474 L476 L477 L526 L527 L528 L529 L562 L565 L566 L567 L622 L623 L624 L625 L658 L661 L662 L663 L712 L713 L714 L715 L748 L751 L752 L753 L808 L809 L810 L811 L844 L847 L848 L849 L899 L900 L901 L902 L903 L906 L907 L940 L943 L944 L945 L983 L984 L985 L986 L987 L990 L991 L993 L1036 L1039 L1040 L1041 L1067 L1068 L1069 L1070 L1071 L1074 L1075 L1077 L1132 L1135 L1136 L1137 L1151 L1152 L1153 L1154 L1155 L1158 L1159 L1161 L1228 L1231 L1232 L1233 L1235 L1236 L1237 L1238 L1239 L1242 L1243 L1245 L1327 L1329 keep common part
extrude "Extrude4" add sketch "Sketch1" along normal blind 69.85
fillet "Fillet1" radius 12.7 4 edges at (196.85, -6.35, 34.925) (196.85, 196.85, 34.925) (-6.35, 196.85, 34.925) (-6.35, -6.35, 34.925)
fillet "Fillet2" radius 6.35 4 edges at (190.5, 190.5, 34.925) (0, 190.5, 34.925) (0, 0, 34.925) (190.5, 0, 34.925)
sketch "Sketch3" plane through (0, 196.85, 0) normal (0, 1, 0) x (-1, 0, 0)
  line L0 (-196.85, 69.85) -> (-184.15, 69.85) construction
  line L1 (-184.15, 69.85) -> (-6.35, 69.85) construction
  line L2 (-196.85, 69.85) -> (-196.85, 0) construction
  line L3 (-184.15, 0) -> (-196.85, 0) construction
  line L4 (-184.15, 0) -> (-6.35, 0) construction
  line L5 (6.35, 0) -> (-6.35, 0) construction
  line L6 (6.35, 0) -> (6.35, 69.85) construction
  line L7 (-6.35, 69.85) -> (6.35, 69.85) construction
  line L8 (6.35, 0) -> (-196.85, 69.85) construction
  line L9 (-196.85, 0) -> (6.35, 69.85) construction
  line L10 (-95.25, 34.925) -> (-75.086, 69.85) construction
  line L11 (-95.25, 34.925) -> (-135.5779, 34.925) construction
  line L12 (-89.7507, 44.45) -> (-100.7493, 44.45)
  line L13 (-100.7493, 44.45) -> (-106.2485, 34.925)
  line L14 (-106.2485, 34.925) -> (-100.7493, 25.4)
  line L15 (-100.7493, 25.4) -> (-89.7507, 25.4)
  line L16 (-89.7507, 25.4) -> (-84.2515, 34.925)
  line L17 (-84.2515, 34.925) -> (-89.7507, 44.45)
  line L18 (-95.25, 34.925) -> (-87.0011, 39.6875) construction
  line L19 (-95.25, 34.925) -> (-103.4989, 39.6875) construction
  line L20 (-378.462, -433.3875) -> (-389.4605, -433.3875)
  line L21 (-389.4605, -433.3875) -> (-394.9597, -442.9125)
  line L22 (-394.9597, -442.9125) -> (-389.4605, -452.4375)
  line L23 (-389.4605, -452.4375) -> (-378.462, -452.4375)
  line L24 (-372.9627, -442.9125) -> (-378.462, -433.3875)
  line L25 (-378.462, -452.4375) -> (-372.9627, -442.9125)
  line L26 (-359.2145, -422.275) -> (-370.2131, -422.275)
  line L27 (-370.2131, -422.275) -> (-375.7123, -431.8)
  line L28 (-375.7123, -431.8) -> (-370.2131, -441.325)
  line L29 (-370.2131, -441.325) -> (-359.2145, -441.325)
  line L30 (-353.7153, -431.8) -> (-359.2145, -422.275)
  line L31 (-359.2145, -441.325) -> (-353.7153, -431.8)
  line L32 (-339.9671, -411.1625) -> (-350.9657, -411.1625)
  line L33 (-350.9657, -411.1625) -> (-356.4649, -420.6875)
  line L34 (-356.4649, -420.6875) -> (-350.9657, -430.2125)
  line L35 (-350.9657, -430.2125) -> (-339.9671, -430.2125)
  line L36 (-334.4679, -420.6875) -> (-339.9671, -411.1625)
  line L37 (-339.9671, -430.2125) -> (-334.4679, -420.6875)
  line L38 (-320.7197, -400.05) -> (-331.7182, -400.05)
  line L39 (-331.7182, -400.05) -> (-337.2175, -409.575)
  line L40 (-337.2175, -409.575) -> (-331.7182, -419.1)
  line L41 (-331.7182, -419.1) -> (-320.7197, -419.1)
  line L42 (-315.2205, -409.575) -> (-320.7197, -400.05)
  line L43 (-320.7197, -419.1) -> (-315.2205, -409.575)
  line L44 (-301.4723, -388.9375) -> (-312.4708, -388.9375)
  line L45 (-312.4708, -388.9375) -> (-317.9701, -398.4625)
  line L46 (-317.9701, -398.4625) -> (-312.4708, -407.9875)
  line L47 (-312.4708, -407.9875) -> (-301.4723, -407.9875)
  line L48 (-295.973, -398.4625) -> (-301.4723, -388.9375)
  line L49 (-301.4723, -407.9875) -> (-295.973, -398.4625)
  line L50 (-282.2249, -377.825) -> (-293.2234, -377.825)
  line L51 (-293.2234, -377.825) -> (-298.7227, -387.35)
  line L52 (-298.7227, -387.35) -> (-293.2234, -396.875)
  line L53 (-293.2234, -396.875) -> (-282.2249, -396.875)
  line L54 (-276.7256, -387.35) -> (-282.2249, -377.825)
  line L55 (-282.2249, -396.875) -> (-276.7256, -387.35)
  line L56 (-262.9775, -366.7125) -> (-273.976, -366.7125)
  line L57 (-273.976, -366.7125) -> (-279.4753, -376.2375)
  line L58 (-279.4753, -376.2375) -> (-273.976, -385.7625)
  line L59 (-273.976, -385.7625) -> (-262.9775, -385.7625)
  line L60 (-257.4782, -376.2375) -> (-262.9775, -366.7125)
  line L61 (-262.9775, -385.7625) -> (-257.4782, -376.2375)
  line L62 (-243.7301, -355.6) -> (-254.7286, -355.6)
  line L63 (-254.7286, -355.6) -> (-260.2278, -365.125)
  line L64 (-260.2278, -365.125) -> (-254.7286, -374.65)
  line L65 (-254.7286, -374.65) -> (-243.7301, -374.65)
  line L66 (-238.2308, -365.125) -> (-243.7301, -355.6)
  line L67 (-243.7301, -374.65) -> (-238.2308, -365.125)
  line L68 (-224.4826, -344.4875) -> (-235.4812, -344.4875)
  line L69 (-235.4812, -344.4875) -> (-240.9804, -354.0125)
  line L70 (-240.9804, -354.0125) -> (-235.4812, -363.5375)
  line L71 (-235.4812, -363.5375) -> (-224.4826, -363.5375)
  line L72 (-218.9834, -354.0125) -> (-224.4826, -344.4875)
  line L73 (-224.4826, -363.5375) -> (-218.9834, -354.0125)
  line L74 (-205.2352, -333.375) -> (-216.2337, -333.375)
  line L75 (-216.2337, -333.375) -> (-221.733, -342.9)
  line L76 (-221.733, -342.9) -> (-216.2337, -352.425)
  line L77 (-216.2337, -352.425) -> (-205.2352, -352.425)
  line L78 (-199.736, -342.9) -> (-205.2352, -333.375)
  line L79 (-205.2352, -352.425) -> (-199.736, -342.9)
  line L80 (-185.9878, -322.2625) -> (-196.9863, -322.2625)
  line L81 (-196.9863, -322.2625) -> (-202.4856, -331.7875)
  line L82 (-202.4856, -331.7875) -> (-196.9863, -341.3125)
  line L83 (-196.9863, -341.3125) -> (-185.9878, -341.3125)
  line L84 (-180.4886, -331.7875) -> (-185.9878, -322.2625)
  line L85 (-185.9878, -341.3125) -> (-180.4886, -331.7875)
  line L86 (-166.7404, -311.15) -> (-177.7389, -311.15)
  line L87 (-177.7389, -311.15) -> (-183.2382, -320.675)
  line L88 (-183.2382, -320.675) -> (-177.7389, -330.2)
  line L89 (-177.7389, -330.2) -> (-166.7404, -330.2)
  line L90 (-161.2411, -320.675) -> (-166.7404, -311.15)
  line L91 (-166.7404, -330.2) -> (-161.2411, -320.675)
  line L92 (-147.493, -300.0375) -> (-158.4915, -300.0375)
  line L93 (-158.4915, -300.0375) -> (-163.9908, -309.5625)
  line L94 (-163.9908, -309.5625) -> (-158.4915, -319.0875)
  line L95 (-158.4915, -319.0875) -> (-147.493, -319.0875)
  line L96 (-141.9937, -309.5625) -> (-147.493, -300.0375)
  line L97 (-147.493, -319.0875) -> (-141.9937, -309.5625)
  line L98 (-128.2456, -288.925) -> (-139.2441, -288.925)
  line L99 (-139.2441, -288.925) -> (-144.7434, -298.45)
  line L100 (-144.7434, -298.45) -> (-139.2441, -307.975)
  line L101 (-139.2441, -307.975) -> (-128.2456, -307.975)
  line L102 (-122.7463, -298.45) -> (-128.2456, -288.925)
  line L103 (-128.2456, -307.975) -> (-122.7463, -298.45)
  line L104 (-108.9982, -277.8125) -> (-119.9967, -277.8125)
  line L105 (-119.9967, -277.8125) -> (-125.4959, -287.3375)
  line L106 (-125.4959, -287.3375) -> (-119.9967, -296.8625)
  line L107 (-119.9967, -296.8625) -> (-108.9982, -296.8625)
  line L108 (-103.4989, -287.3375) -> (-108.9982, -277.8125)
  line L109 (-108.9982, -296.8625) -> (-103.4989, -287.3375)
  line L110 (-89.7507, -266.7) -> (-100.7493, -266.7)
  line L111 (-100.7493, -266.7) -> (-106.2485, -276.225)
  line L112 (-106.2485, -276.225) -> (-100.7493, -285.75)
  line L113 (-100.7493, -285.75) -> (-89.7507, -285.75)
  line L114 (-84.2515, -276.225) -> (-89.7507, -266.7)
  line L115 (-89.7507, -285.75) -> (-84.2515, -276.225)
  line L116 (-70.5033, -255.5875) -> (-81.5018, -255.5875)
  line L117 (-81.5018, -255.5875) -> (-87.0011, -265.1125)
  line L118 (-87.0011, -265.1125) -> (-81.5018, -274.6375)
  line L119 (-81.5018, -274.6375) -> (-70.5033, -274.6375)
  line L120 (-65.0041, -265.1125) -> (-70.5033, -255.5875)
  line L121 (-70.5033, -274.6375) -> (-65.0041, -265.1125)
  line L122 (-51.2559, -244.475) -> (-62.2544, -244.475)
  line L123 (-62.2544, -244.475) -> (-67.7537, -254)
  line L124 (-67.7537, -254) -> (-62.2544, -263.525)
  line L125 (-62.2544, -263.525) -> (-51.2559, -263.525)
  line L126 (-45.7566, -254) -> (-51.2559, -244.475)
  line L127 (-51.2559, -263.525) -> (-45.7566, -254)
  line L128 (-32.0085, -233.3625) -> (-43.007, -233.3625)
  line L129 (-43.007, -233.3625) -> (-48.5063, -242.8875)
  line L130 (-48.5063, -242.8875) -> (-43.007, -252.4125)
  line L131 (-43.007, -252.4125) -> (-32.0085, -252.4125)
  line L132 (-26.5092, -242.8875) -> (-32.0085, -233.3625)
  line L133 (-32.0085, -252.4125) -> (-26.5092, -242.8875)
  line L134 (-12.7611, -222.25) -> (-23.7596, -222.25)
  line L135 (-23.7596, -222.25) -> (-29.2589, -231.775)
  line L136 (-29.2589, -231.775) -> (-23.7596, -241.3)
  line L137 (-23.7596, -241.3) -> (-12.7611, -241.3)
  line L138 (-7.2618, -231.775) -> (-12.7611, -222.25)
  line L139 (-12.7611, -241.3) -> (-7.2618, -231.775)
  line L140 (6.4863, -211.1375) -> (-4.5122, -211.1375)
  line L141 (-4.5122, -211.1375) -> (-10.0114, -220.6625)
  line L142 (-10.0114, -220.6625) -> (-4.5122, -230.1875)
  line L143 (-4.5122, -230.1875) -> (6.4863, -230.1875)
  line L144 (11.9856, -220.6625) -> (6.4863, -211.1375)
  line L145 (6.4863, -230.1875) -> (11.9856, -220.6625)
  line L146 (25.7337, -200.025) -> (14.7352, -200.025)
  line L147 (14.7352, -200.025) -> (9.236, -209.55)
  line L148 (9.236, -209.55) -> (14.7352, -219.075)
  line L149 (14.7352, -219.075) -> (25.7337, -219.075)
  line L150 (31.233, -209.55) -> (25.7337, -200.025)
  line L151 (25.7337, -219.075) -> (31.233, -209.55)
  line L152 (44.9812, -188.9125) -> (33.9826, -188.9125)
  line L153 (33.9826, -188.9125) -> (28.4834, -198.4375)
  line L154 (28.4834, -198.4375) -> (33.9826, -207.9625)
  line L155 (33.9826, -207.9625) -> (44.9812, -207.9625)
  line L156 (50.4804, -198.4375) -> (44.9812, -188.9125)
  line L157 (44.9812, -207.9625) -> (50.4804, -198.4375)
  line L158 (64.2286, -177.8) -> (53.2301, -177.8)
  line L159 (53.2301, -177.8) -> (47.7308, -187.325)
  line L160 (47.7308, -187.325) -> (53.2301, -196.85)
  line L161 (53.2301, -196.85) -> (64.2286, -196.85)
  line L162 (69.7278, -187.325) -> (64.2286, -177.8)
  line L163 (64.2286, -196.85) -> (69.7278, -187.325)
  line L164 (83.476, -166.6875) -> (72.4775, -166.6875)
  line L165 (72.4775, -166.6875) -> (66.9782, -176.2125)
  line L166 (66.9782, -176.2125) -> (72.4775, -185.7375)
  line L167 (72.4775, -185.7375) -> (83.476, -185.7375)
  line L168 (88.9753, -176.2125) -> (83.476, -166.6875)
  line L169 (83.476, -185.7375) -> (88.9753, -176.2125)
  line L170 (102.7234, -155.575) -> (91.7249, -155.575)
  line L171 (91.7249, -155.575) -> (86.2256, -165.1)
  line L172 (86.2256, -165.1) -> (91.7249, -174.625)
  line L173 (91.7249, -174.625) -> (102.7234, -174.625)
  line L174 (108.2227, -165.1) -> (102.7234, -155.575)
  line L175 (102.7234, -174.625) -> (108.2227, -165.1)
  line L176 (121.9708, -144.4625) -> (110.9723, -144.4625)
  line L177 (110.9723, -144.4625) -> (105.473, -153.9875)
  line L178 (105.473, -153.9875) -> (110.9723, -163.5125)
  line L179 (110.9723, -163.5125) -> (121.9708, -163.5125)
  line L180 (127.4701, -153.9875) -> (121.9708, -144.4625)
  line L181 (121.9708, -163.5125) -> (127.4701, -153.9875)
  line L182 (141.2182, -133.35) -> (130.2197, -133.35)
  line L183 (130.2197, -133.35) -> (124.7205, -142.875)
  line L184 (124.7205, -142.875) -> (130.2197, -152.4)
  line L185 (130.2197, -152.4) -> (141.2182, -152.4)
  line L186 (146.7175, -142.875) -> (141.2182, -133.35)
  line L187 (141.2182, -152.4) -> (146.7175, -142.875)
  line L188 (160.4657, -122.2375) -> (149.4671, -122.2375)
  line L189 (149.4671, -122.2375) -> (143.9679, -131.7625)
  line L190 (143.9679, -131.7625) -> (149.4671, -141.2875)
  line L191 (149.4671, -141.2875) -> (160.4657, -141.2875)
  line L192 (165.9649, -131.7625) -> (160.4657, -122.2375)
  line L193 (160.4657, -141.2875) -> (165.9649, -131.7625)
  line L194 (179.7131, -111.125) -> (168.7145, -111.125)
  line L195 (168.7145, -111.125) -> (163.2153, -120.65)
  line L196 (163.2153, -120.65) -> (168.7145, -130.175)
  line L197 (168.7145, -130.175) -> (179.7131, -130.175)
  line L198 (185.2123, -120.65) -> (179.7131, -111.125)
  line L199 (179.7131, -130.175) -> (185.2123, -120.65)
  line L200 (198.9605, -100.0125) -> (187.962, -100.0125)
  line L201 (187.962, -100.0125) -> (182.4627, -109.5375)
  line L202 (182.4627, -109.5375) -> (187.962, -119.0625)
  line L203 (187.962, -119.0625) -> (198.9605, -119.0625)
  line L204 (204.4597, -109.5375) -> (198.9605, -100.0125)
  line L205 (198.9605, -119.0625) -> (204.4597, -109.5375)
  line L206 (218.2079, -88.9) -> (207.2094, -88.9)
  line L207 (207.2094, -88.9) -> (201.7101, -98.425)
  line L208 (201.7101, -98.425) -> (207.2094, -107.95)
  line L209 (207.2094, -107.95) -> (218.2079, -107.95)
  line L210 (223.7072, -98.425) -> (218.2079, -88.9)
  line L211 (218.2079, -107.95) -> (223.7072, -98.425)
  line L212 (237.4553, -77.7875) -> (226.4568, -77.7875)
  line L213 (226.4568, -77.7875) -> (220.9575, -87.3125)
  line L214 (220.9575, -87.3125) -> (226.4568, -96.8375)
  line L215 (226.4568, -96.8375) -> (237.4553, -96.8375)
  line L216 (242.9546, -87.3125) -> (237.4553, -77.7875)
  line L217 (237.4553, -96.8375) -> (242.9546, -87.3125)
  line L218 (256.7027, -66.675) -> (245.7042, -66.675)
  line L219 (245.7042, -66.675) -> (240.2049, -76.2)
  line L220 (240.2049, -76.2) -> (245.7042, -85.725)
  line L221 (245.7042, -85.725) -> (256.7027, -85.725)
  line L222 (262.202, -76.2) -> (256.7027, -66.675)
  line L223 (256.7027, -85.725) -> (262.202, -76.2)
  line L224 (275.9501, -55.5625) -> (264.9516, -55.5625)
  line L225 (264.9516, -55.5625) -> (259.4524, -65.0875)
  line L226 (259.4524, -65.0875) -> (264.9516, -74.6125)
  line L227 (264.9516, -74.6125) -> (275.9501, -74.6125)
  line L228 (281.4494, -65.0875) -> (275.9501, -55.5625)
  line L229 (275.9501, -74.6125) -> (281.4494, -65.0875)
  line L230 (295.1976, -44.45) -> (284.199, -44.45)
  line L231 (284.199, -44.45) -> (278.6998, -53.975)
  line L232 (278.6998, -53.975) -> (284.199, -63.5)
  line L233 (284.199, -63.5) -> (295.1976, -63.5)
  line L234 (300.6968, -53.975) -> (295.1976, -44.45)
  line L235 (295.1976, -63.5) -> (300.6968, -53.975)
  line L236 (314.445, -33.3375) -> (303.4464, -33.3375)
  line L237 (303.4464, -33.3375) -> (297.9472, -42.8625)
  line L238 (297.9472, -42.8625) -> (303.4464, -52.3875)
  line L239 (303.4464, -52.3875) -> (314.445, -52.3875)
  line L240 (319.9442, -42.8625) -> (314.445, -33.3375)
  line L241 (314.445, -52.3875) -> (319.9442, -42.8625)
  line L242 (333.6924, -22.225) -> (322.6939, -22.225)
  line L243 (322.6939, -22.225) -> (317.1946, -31.75)
  line L244 (317.1946, -31.75) -> (322.6939, -41.275)
  line L245 (322.6939, -41.275) -> (333.6924, -41.275)
  line L246 (339.1916, -31.75) -> (333.6924, -22.225)
  line L247 (333.6924, -41.275) -> (339.1916, -31.75)
  line L248 (352.9398, -11.1125) -> (341.9413, -11.1125)
  line L249 (341.9413, -11.1125) -> (336.442, -20.6375)
  line L250 (336.442, -20.6375) -> (341.9413, -30.1625)
  line L251 (341.9413, -30.1625) -> (352.9398, -30.1625)
  line L252 (358.4391, -20.6375) -> (352.9398, -11.1125)
  line L253 (352.9398, -30.1625) -> (358.4391, -20.6375)
  line L254 (372.1872, 0) -> (361.1887, 0)
  line L255 (361.1887, 0) -> (355.6894, -9.525)
  line L256 (355.6894, -9.525) -> (361.1887, -19.05)
  line L257 (361.1887, -19.05) -> (372.1872, -19.05)
  line L258 (377.6865, -9.525) -> (372.1872, 0)
  line L259 (372.1872, -19.05) -> (377.6865, -9.525)
  line L260 (391.4346, 11.1125) -> (380.4361, 11.1125)
  line L261 (380.4361, 11.1125) -> (374.9368, 1.5875)
  line L262 (374.9368, 1.5875) -> (380.4361, -7.9375)
  line L263 (380.4361, -7.9375) -> (391.4346, -7.9375)
  line L264 (396.9339, 1.5875) -> (391.4346, 11.1125)
  line L265 (391.4346, -7.9375) -> (396.9339, 1.5875)
  line L266 (410.682, 22.225) -> (399.6835, 22.225)
  line L267 (399.6835, 22.225) -> (394.1843, 12.7)
  line L268 (394.1843, 12.7) -> (399.6835, 3.175)
  line L269 (399.6835, 3.175) -> (410.682, 3.175)
  line L270 (416.1813, 12.7) -> (410.682, 22.225)
  line L271 (410.682, 3.175) -> (416.1813, 12.7)
  line L272 (429.9295, 33.3375) -> (418.9309, 33.3375)
  line L273 (418.9309, 33.3375) -> (413.4317, 23.8125)
  line L274 (413.4317, 23.8125) -> (418.9309, 14.2875)
  line L275 (418.9309, 14.2875) -> (429.9295, 14.2875)
  line L276 (435.4287, 23.8125) -> (429.9295, 33.3375)
  line L277 (429.9295, 14.2875) -> (435.4287, 23.8125)
  line L278 (449.1769, 44.45) -> (438.1783, 44.45)
  line L279 (438.1783, 44.45) -> (432.6791, 34.925)
  line L280 (432.6791, 34.925) -> (438.1783, 25.4)
  line L281 (438.1783, 25.4) -> (449.1769, 25.4)
  line L282 (454.6761, 34.925) -> (449.1769, 44.45)
  line L283 (449.1769, 25.4) -> (454.6761, 34.925)
  line L284 (468.4243, 55.5625) -> (457.4258, 55.5625)
  line L285 (457.4258, 55.5625) -> (451.9265, 46.0375)
  line L286 (451.9265, 46.0375) -> (457.4258, 36.5125)
  line L287 (457.4258, 36.5125) -> (468.4243, 36.5125)
  line L288 (473.9235, 46.0375) -> (468.4243, 55.5625)
  line L289 (468.4243, 36.5125) -> (473.9235, 46.0375)
  line L290 (487.6717, 66.675) -> (476.6732, 66.675)
  line L291 (476.6732, 66.675) -> (471.1739, 57.15)
  line L292 (471.1739, 57.15) -> (476.6732, 47.625)
  line L293 (476.6732, 47.625) -> (487.6717, 47.625)
  line L294 (493.171, 57.15) -> (487.6717, 66.675)
  line L295 (487.6717, 47.625) -> (493.171, 57.15)
  line L296 (506.9191, 77.7875) -> (495.9206, 77.7875)
  line L297 (495.9206, 77.7875) -> (490.4213, 68.2625)
  line L298 (490.4213, 68.2625) -> (495.9206, 58.7375)
  line L299 (495.9206, 58.7375) -> (506.9191, 58.7375)
  line L300 (512.4184, 68.2625) -> (506.9191, 77.7875)
  line L301 (506.9191, 58.7375) -> (512.4184, 68.2625)
  line L302 (526.1665, 88.9) -> (515.168, 88.9)
  line L303 (515.168, 88.9) -> (509.6687, 79.375)
  line L304 (509.6687, 79.375) -> (515.168, 69.85)
  line L305 (515.168, 69.85) -> (526.1665, 69.85)
  line L306 (531.6658, 79.375) -> (526.1665, 88.9)
  line L307 (526.1665, 69.85) -> (531.6658, 79.375)
  line L308 (545.4139, 100.0125) -> (534.4154, 100.0125)
  line L309 (534.4154, 100.0125) -> (528.9162, 90.4875)
  line L310 (528.9162, 90.4875) -> (534.4154, 80.9625)
  line L311 (534.4154, 80.9625) -> (545.4139, 80.9625)
  line L312 (550.9132, 90.4875) -> (545.4139, 100.0125)
  line L313 (545.4139, 80.9625) -> (550.9132, 90.4875)
  line L314 (564.6614, 111.125) -> (553.6628, 111.125)
  line L315 (553.6628, 111.125) -> (548.1636, 101.6)
  line L316 (548.1636, 101.6) -> (553.6628, 92.075)
  line L317 (553.6628, 92.075) -> (564.6614, 92.075)
  line L318 (570.1606, 101.6) -> (564.6614, 111.125)
  line L319 (564.6614, 92.075) -> (570.1606, 101.6)
  line L320 (583.9088, 122.2375) -> (572.9102, 122.2375)
  line L321 (572.9102, 122.2375) -> (567.411, 112.7125)
  line L322 (567.411, 112.7125) -> (572.9102, 103.1875)
  line L323 (572.9102, 103.1875) -> (583.9088, 103.1875)
  line L324 (589.408, 112.7125) -> (583.9088, 122.2375)
  line L325 (583.9088, 103.1875) -> (589.408, 112.7125)
  line L326 (603.1562, 133.35) -> (592.1577, 133.35)
  line L327 (592.1577, 133.35) -> (586.6584, 123.825)
  line L328 (586.6584, 123.825) -> (592.1577, 114.3)
  line L329 (592.1577, 114.3) -> (603.1562, 114.3)
  line L330 (608.6554, 123.825) -> (603.1562, 133.35)
  line L331 (603.1562, 114.3) -> (608.6554, 123.825)
  line L332 (622.4036, 144.4625) -> (611.4051, 144.4625)
  line L333 (611.4051, 144.4625) -> (605.9058, 134.9375)
  line L334 (605.9058, 134.9375) -> (611.4051, 125.4125)
  line L335 (611.4051, 125.4125) -> (622.4036, 125.4125)
  line L336 (627.9029, 134.9375) -> (622.4036, 144.4625)
  line L337 (622.4036, 125.4125) -> (627.9029, 134.9375)
  line L338 (641.651, 155.575) -> (630.6525, 155.575)
  line L339 (630.6525, 155.575) -> (625.1532, 146.05)
  line L340 (625.1532, 146.05) -> (630.6525, 136.525)
  line L341 (630.6525, 136.525) -> (641.651, 136.525)
  line L342 (647.1503, 146.05) -> (641.651, 155.575)
  line L343 (641.651, 136.525) -> (647.1503, 146.05)
  line L344 (660.8984, 166.6875) -> (649.8999, 166.6875)
  line L345 (649.8999, 166.6875) -> (644.4006, 157.1625)
  line L346 (644.4006, 157.1625) -> (649.8999, 147.6375)
  line L347 (649.8999, 147.6375) -> (660.8984, 147.6375)
  line L348 (666.3977, 157.1625) -> (660.8984, 166.6875)
  line L349 (660.8984, 147.6375) -> (666.3977, 157.1625)
  line L350 (680.1458, 177.8) -> (669.1473, 177.8)
  line L351 (669.1473, 177.8) -> (663.6481, 168.275)
  line L352 (663.6481, 168.275) -> (669.1473, 158.75)
  line L353 (669.1473, 158.75) -> (680.1458, 158.75)
  line L354 (685.6451, 168.275) -> (680.1458, 177.8)
  line L355 (680.1458, 158.75) -> (685.6451, 168.275)
  line L356 (699.3933, 188.9125) -> (688.3947, 188.9125)
  line L357 (688.3947, 188.9125) -> (682.8955, 179.3875)
  line L358 (682.8955, 179.3875) -> (688.3947, 169.8625)
  line L359 (688.3947, 169.8625) -> (699.3933, 169.8625)
  line L360 (704.8925, 179.3875) -> (699.3933, 188.9125)
  line L361 (699.3933, 169.8625) -> (704.8925, 179.3875)